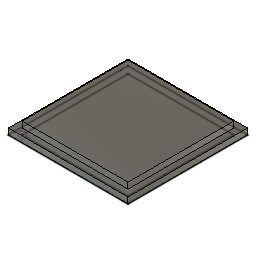
adaptor lid final (Autodesk Fusion 360 design; units mm, degrees)
Autodesk Fusion 360 part; units mm, degrees
sketch "Sketch1" plane through (0, 0, 0) normal (0, 0, 1) x (1, 0, 0)
  line L0 (0, 0) -> (177, 0)
  line L1 (177, 0) -> (177, 177)
  line L2 (177, 177) -> (0, 177)
  line L3 (0, 177) -> (0, 0)
  line L4 (-11.5, 177) -> (-11.5, -11.5)
  line L5 (-11.5, -11.5) -> (180, -11.5)
  line L6 (188.5, 188.5) -> (188.5, -11.5)
  line L7 (180, -11.5) -> (188.5, -11.5)
  line L8 (188.5, 188.5) -> (-11.5, 188.5)
  line L9 (-11.5, 177) -> (-11.5, 188.5)
  dimension "d1" = 177
  dimension "d2" = 177
  dimension "d3" = 11.5
  dimension "d4" = 11.5
  dimension "d5" = 11.5
  dimension "d6" = 11.5
  constraint horizontal L0
  constraint vertical L1
  constraint horizontal L2
  constraint vertical L3
  constraint coincident L0.start L3.end
  constraint parallel L3 L4
  constraint perpendicular L4 L5
  constraint perpendicular L5 L6
  constraint perpendicular L6 L7
  constraint perpendicular L6 L8
  constraint perpendicular L8 L9
  measures "d1" distance of L0.start L2.end
  measures "d2" distance of L0.start L0.end
  measures "d3" distance of L3 L4
  measures "d4" distance of L0 L5
  measures "d5" distance of L1 L6
  measures "d6" distance of L2 L8
extrude "Extrude1" add sketch "Sketch1" along normal blind 20 contours L0 L1 L2 L3
extrude "Extrude2" add sketch "Sketch1" along normal blind 10
